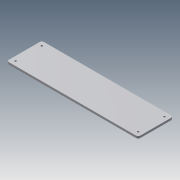
# Autodesk Inventor part: ProjectorPlateBack
Saved by Autodesk Inventor 2014 (Build 180170000, 170)
## iProperties
Created: 2014-08-10
Part Number: ProjectorPlateBack
Material: Generic
Document SubType Name: Modeling
Designer: Peele
Density: 1 g/cm^3
Appearance: White
Author: Peele
Autodesk Inventor part; units mm, degrees
ref_plane "YZ Plane" through (0, 0, 0) normal (1, 0, 0) x (0, 1, 0)
ref_plane "XZ Plane" through (0, 0, 0) normal (0, 1, 0) x (-1, 0, 0)
ref_plane "XY Plane" through (0, 0, 0) normal (0, 0, 1) x (1, 0, 0)
sketch "Sketch1" plane through (0, 0, 0) normal (0, 0, 1) x (1, 0, 0)
  line L0 (-187.5, -50) -> (187.5, -50)
  line L1 (187.5, -50) -> (187.5, 50)
  line L2 (187.5, 50) -> (-187.5, 50)
  line L3 (-187.5, 50) -> (-187.5, -50)
  line L4 (-187.5, -50) -> (187.5, 50) construction
  line L5 (187.5, -50) -> (-187.5, 50) construction
  point P0 (0, 0)
  dimension "d0" = 375
  dimension "d1" = 100
  constraints: 12 end point, 2 midpoint, 2 parallel, 1 horizontal, 1 perpendicular
  measures "d0" distance of L0.start L0.end
  measures "d1" distance of L0.end L1.end
extrude "Extrusion1" add sketch "Sketch1" along normal blind 6
sketch "Sketch8" plane through (0, 0, 6) normal (0, 0, 1) x (1, 0, 0)
  circle A0 centre (-175, 37.5) radius 2.7
  circle A1 centre (-175, -37.5) radius 2.7
  circle A2 centre (175, -37.5) radius 2.7
  circle A3 centre (175, 37.5) radius 2.7
  line L0 (-187.5, 50) -> (-187.5, -50) projected
  line L1 (187.5, 50) -> (-187.5, 50) projected
  line L2 (187.5, -50) -> (187.5, 50) projected
  line L3 (-187.5, -50) -> (187.5, -50) projected
  dimension "d40" = 12.5
  dimension "d41" = 12.5
  dimension "d42" = 12.5
  dimension "d43" = 12.5
  dimension "d44" = 5.4
  constraints: 4 centre point, 3 equal radius, 2 horizontal alignment, 2 vertical alignment
  measures "d40" distance from line of L0 A0.centre
  measures "d41" distance from line of A0.centre L1
  measures "d42" distance from line of A2.centre L2
  measures "d43" distance from line of A2.centre L3
  measures "d44" diameter of A0
extrude "Extrusion8" cut sketch "Sketch8" against normal through all contours A0 | A1 | A2 | A3
fillet "Fillet3" radius 6 4 edges at (187.5, -50, 3) (-187.5, 50, 3) (-187.5, -50, 3) (187.5, 50, 3)
equation "\"d41\" = d40"
equation "\"d42\" = d40"
equation "\"d43\" = d40"
body "Solid1"
